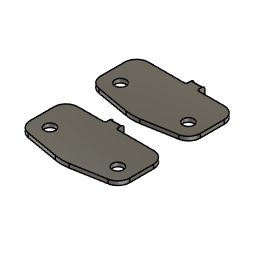
Securite_porte (Autodesk Fusion 360 design; units mm, degrees)
Autodesk Fusion 360 part; units mm, degrees
sketch "Sketch1" plane through (0, 0, 0) normal (0, 0, 1) x (1, 0, 0)
  line L0 (0, 0) -> (50.1, 0)
  line L1 (50.1, 0) -> (50.1, 27.5)
  line L2 (0, 27.5) -> (0, 0)
  circle A0 centre (7.96, 11.45) radius 2.75
  circle A1 centre (42.14, 11.45) radius 2.75
  line L3 (25.2, 27.5) -> (25.2, 31)
  line L4 (25.2, 31) -> (19.7, 31)
  line L5 (19.7, 31) -> (19.7, 27.5)
  line L6 (50.1, 27.5) -> (25.2, 27.5)
  line L7 (19.7, 27.5) -> (0, 27.5)
  line L8 (19.7, 27.5) -> (25.552, 27.5)
  line L9 (25.05, 0) -> (50.1, 4.417)
  line L10 (25.05, 0) -> (50, 0) construction
  line L11 (25.05, 0) -> (0, 4.417)
  line L12 (25.05, 0) -> (0, 0) construction
  dimension "d1" = 50.1
  dimension "d2" = 27.5
  dimension "d3" = 5.5
  dimension "d4" = 5.5
  dimension "d6" = 7.96
  dimension "d7" = 7.96
  dimension "d10" = 5.5
  dimension "d11" = 3.5
  dimension "d19" = 10
  dimension "d20" = 10
  dimension "d26" = 16.05
  dimension "d27" = 16.05
  dimension "d38" = 30.4
  dimension "d39" = 25.2
  constraint horizontal L0
  constraint vertical L1
  constraint horizontal L6
  constraint vertical L2
  constraint coincident L0.start L2.end
  constraint vertical L3
  constraint horizontal L4
  constraint vertical L5
  constraint coincident L5.end L6
  constraint collinear L6 L7
  constraint coincident L6 L8.end
  constraint perpendicular L3 L8
  constraint midpoint L0 L9.start
  constraint horizontal L10
  constraint horizontal L12
  constraint coincident L1 L9.end
  constraint coincident L2 L11.end
  measures "d1" distance of L0.start L0.end
  measures "d2" distance of L0.start L2.start
  measures "d3" diameter of A0
  measures "d4" diameter of A1
  measures "d6" distance of L2 A0.centre
  measures "d7" distance of L1 A1.centre
  measures "d10" distance of L5.end L3.start
  measures "d11" distance of L5.end L4.end
  measures "d19" angle of L9 L10
  measures "d20" angle of L11 L12
  measures "d26" distance of A0.centre L7
  measures "d27" distance of A1.centre L6
  measures "d38" distance of L1 L5
  measures "d39" distance of L2 L3
extrude "Extrude2" add sketch "Sketch1" along normal blind 2 contours L3 L4 L5 L8 makes body 1
extrude "Extrude3" add sketch "Sketch1" along normal blind 2 separate body contours L1 L2 L6 L7 L8 L9 L11 | L3 L4 L5 L8 makes body 2
fillet "Fillet1" radius 20 1 edges at (25.05, 0, 1) on bodies 2
fillet "Fillet2" radius 6 4 edges at (50.1, 4.417, 1) (0, 4.417, 1) (50.1, 27.5, 1) (0, 27.5, 1) on bodies 2
extrude "Extrude4" add sketch "Sketch1" against normal blind 5.3 contours L3 L4 L5 L8 bodies 1 2
fillet "Fillet3" radius 1.5 1 edges at (22.45, 31, 2) on bodies 1
fillet "Fillet4" radius 0.5 1 edges at (22.45, 27.5, 0) on bodies 1
fillet "Fillet5" radius 1 2 edges at (19.7, 27.5, 1) (25.2, 27.5, 1) on bodies 1
delete_face "DeleteFace1" 1 faces at (23.3667, 29.5714, 1.9983) on bodies 1
extrude "Extrude5" add 1 faces at (23.3667, 31, -2.8667) along direction (0, 1, 0) blind 0.5 on bodies 1 bodies 1
fillet "Fillet6" radius 1.5 1 edges at (22.45, 31.5, 2) on bodies 1
delete_face "DeleteFace2" 1 faces at (21.5333, 27.345, -0.1381) on bodies 1
fillet "Fillet7" radius 1.25 1 edges at (22.45, 27.5, 0) on bodies 1
mirror "Mirror1" about plane through (0, 0, 0) normal (1, 0, 0) of bodies 1 makes body 3
move_body "Move1" bodies 3 to x (1, 0, 0) y (0, 1, 0) z (0, 0, 1) at (48.4289, 37.2018, 0)
equation "d6 = 5.21 mm + ( 5.5 / 2 ) * 1 mm"
equation "d7 = 5.21 mm + ( 5.5 / 2 ) * 1 mm"
equation "d26 = 13.3 mm + ( 5.5 / 2 ) * 1 mm"
